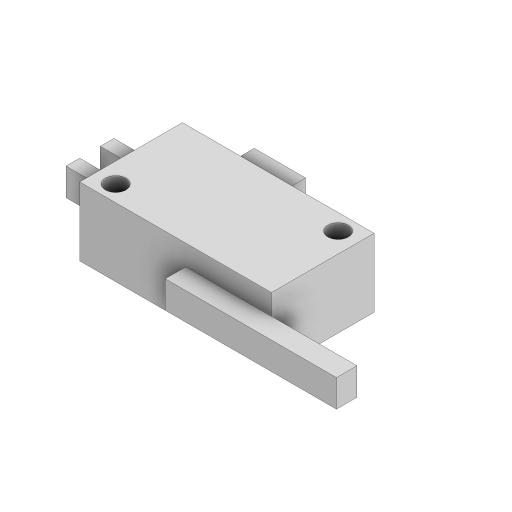
# Autodesk Inventor part: FINAL_DE_CARRERA
Saved by Autodesk Inventor 2024 (Build 280153000, 153)
## iProperties
Created: 2024-08-21
Part Number: FINAL_DE_CARRERA
Material: Generic
Document SubType Name: Modeling
Designer: Jhuliams
Density: 1 g/cm^3
Appearance: Default
Author: Jhuliams
Autodesk Inventor part; units mm, degrees
ref_plane "YZ Plane" through (0, 0, 0) normal (1, 0, 0) x (0, 1, 0)
ref_plane "XZ Plane" through (0, 0, 0) normal (0, 1, 0) x (-1, 0, 0)
ref_plane "XY Plane" through (0, 0, 0) normal (0, 0, 1) x (1, 0, 0)
sketch "Sketch1" plane through (0, 0, 0) normal (0, 1, 0) x (-1, 0, 0)
  line L0 (14, 7.5) -> (-14, 7.5)
  line L1 (-14, 7.5) -> (-14, -7.5)
  line L2 (-14, -7.5) -> (14, -7.5)
  line L3 (14, -7.5) -> (14, 7.5)
  line L4 (14, 7.5) -> (-14, -7.5) construction
  line L5 (-14, 7.5) -> (14, -7.5) construction
  point P0 (0, 0)
  dimension "d0" = 28
  dimension "d1" = 15
  constraints: 12 end point, 2 midpoint, 2 parallel, 1 horizontal, 1 perpendicular
  measures "d0" distance of L2.end L1.end
  measures "d1" distance of L1.end L0.end
extrude "Extrusion1" add sketch "Sketch1" along normal blind 10
sketch "Sketch2" plane through (-14, 0, 7.5) normal (0, 0, 1) x (1, 0, 0)
  line L0 (15.5, 7) -> (40.5, 7)
  line L1 (40.5, 7) -> (40.5, 3)
  line L2 (40.5, 3) -> (15.5, 3)
  line L3 (15.5, 3) -> (15.5, 7)
  line L4 (28, 0) -> (28, 10) projected
  line L5 (15.5, 7) -> (40.5, 3) construction
  line L6 (40.5, 7) -> (15.5, 3) construction
  point P0 (14, 0)
  point P1 (28, 5)
  dimension "d4" = 25
  dimension "d5" = 4
  constraints: 12 end point, 3 midpoint, 2 parallel, 1 horizontal, 1 perpendicular
  measures "d4" distance of L1.end L2.end
  measures "d5" distance of L0.end L1.end
extrude "Extrusion2" add sketch "Sketch2" along normal blind 3
sketch "Sketch3" plane through (14, 0, -7.5) normal (0, 0, -1) x (-1, 0, 0)
  line L0 (0, 3) -> (0, 7) projected
  line L1 (0, 5) -> (15, 5)
  line L2 (16.5, 3) -> (13.5, 3)
  line L3 (13.5, 3) -> (13.5, 7)
  line L4 (13.5, 7) -> (16.5, 7)
  line L5 (16.5, 7) -> (16.5, 3)
  line L6 (16.5, 3) -> (13.5, 7) construction
  line L7 (13.5, 3) -> (16.5, 7) construction
  line L8 (15, 3) -> (15, 7)
  point P0 (14, 0)
  dimension "d8" = 15
  dimension "d9" = 3
  constraints: 16 end point, 5 midpoint, 2 horizontal, 2 parallel, 1 perpendicular
  measures "d8" distance of L1.start L1.end
  measures "d9" distance of L3.end L4.end
extrude "Extrusion3" add sketch "Sketch3" along normal blind 5 contours L8 L4 L5 L2
sketch "Sketch4" plane through (-2.5, 3, -7.5) normal (-1, 0, 0) x (0, 0, 1)
  line L0 (-5, 4) -> (-5, 0) projected
  line L1 (-5, 4) -> (-3, 4)
  line L2 (-3, 4) -> (-3, 0)
  line L3 (-3, 0) -> (-5, 0)
  line L4 (-5, 0) -> (-5, 4)
  point P0 (7.5, -3)
  dimension "d12" = 2
  constraints: 8 end point, 2 parallel, 1 horizontal, 1 perpendicular
  measures "d12" distance of L2.end L3.end
extrude "Extrusion4" add sketch "Sketch4" along normal blind 6
sketch "Sketch5" plane through (-14, 0, -7.5) normal (-1, 0, 0) x (0, 0, 1)
  line L0 (0, 0) -> (0, 10) projected
  line L1 (0, 5) -> (4, 5)
  line L2 (6, 3) -> (2, 3)
  line L3 (2, 3) -> (2, 7)
  line L4 (2, 7) -> (6, 7)
  line L5 (6, 7) -> (6, 3)
  line L6 (6, 3) -> (2, 7) construction
  line L7 (2, 3) -> (6, 7) construction
  line L8 (4, 3) -> (4, 7)
  line L9 (7.5, 0) -> (7.5, 3)
  line L10 (15, 5) -> (11, 5)
  line L11 (9, 3) -> (13, 3)
  line L12 (13, 3) -> (13, 7)
  line L13 (13, 7) -> (9, 7)
  line L14 (9, 7) -> (9, 3)
  line L15 (9, 3) -> (13, 7) construction
  line L16 (13, 3) -> (9, 7) construction
  line L17 (11, 3) -> (11, 7)
  dimension "d15" = 4
  dimension "d16" = 4
  dimension "d17" = 4
  dimension "d18" = 3
  constraints: 34 end point, 8 symmetric about line, 5 midpoint, 2 horizontal, 2 parallel, 1 perpendicular, 1 vertical
  measures "d15" distance of L1.start L1.end
  measures "d16" distance of L3.end L4.end
  measures "d17" distance of L2.end L3.end
  measures "d18" distance of L9.start L9.end
extrude "Extrusion5" add sketch "Sketch5" along normal blind 6 contours L8 L4 L5 L2 | L17 L11 L14 L13
sketch "Sketch7" plane through (0, 0, 0) normal (0, -1, 0) x (1, 0, 0)
  line L0 (14, 7.5) -> (14, -7.5) projected
  line L1 (-14, -7.5) -> (-14, 7.5) projected
  line L2 (11.1, -5.15) -> (-11.1, -5.15)
  line L3 (-11.1, -5.15) -> (-11.1, 5.15)
  line L4 (-11.1, 5.15) -> (11.1, 5.15)
  line L5 (11.1, 5.15) -> (11.1, -5.15)
  line L6 (11.1, -5.15) -> (-11.1, 5.15) construction
  line L7 (-11.1, -5.15) -> (11.1, 5.15) construction
  circle A0 centre (-11.1, 5.15) radius 1.5
  circle A1 centre (11.1, -5.15) radius 1.5
  point P0 (0, 0)
  dimension "d40" = 22.2
  dimension "d41" = 10.3
  dimension "d42" = 3
  dimension "d43" = 3
  constraints: 12 end point, 2 centre point, 2 coincident, 2 midpoint, 2 parallel, 1 horizontal, 1 perpendicular
  measures "d40" distance of L3.end L4.end
  measures "d41" distance of L2.end L3.end
  measures "d42" diameter of A0
  measures "d43" diameter of A1
extrude "Extrusion7" cut sketch "Sketch7" against normal blind 15 contours L5 A1 L2 | L2 A1 L5 | A0 L4 L3 | L3 L4 A0
body "Solid1"
